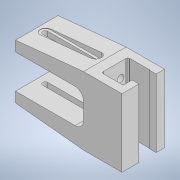
# Autodesk Inventor part: Z Belt 2
Saved by Autodesk Inventor 2022 (Build 260153000, 153)
## iProperties
Created: 2022-02-24
Part Number: Z Belt 2
Material: Generic
Document SubType Name: Modeling
Designer: Nicoli
Density: 1 g/cm^3
Appearance: Default
Author: Nicoli
Autodesk Inventor part; units mm, degrees
ref_plane "YZ Plane" through (0, 0, 0) normal (1, 0, 0) x (0, 1, 0)
ref_plane "XZ Plane" through (0, 0, 0) normal (0, 1, 0) x (-1, 0, 0)
ref_plane "XY Plane" through (0, 0, 0) normal (0, 0, 1) x (1, 0, 0)
sketch "Sketch1" plane through (0, 0, 0) normal (0, 0, 1) x (1, 0, 0)
  line L0 (-40, 0) -> (0, 0)
  line L1 (0, 0) -> (0, -20)
  line L2 (0, -20) -> (-40, -20)
  line L3 (-40, -20) -> (-40, -26)
  line L4 (-40, -26) -> (0, -30)
  line L5 (0, -30) -> (6, -30)
  line L6 (6, -30) -> (6, 10)
  line L7 (6, 10) -> (0, 10)
  line L8 (0, 10) -> (-40, 6)
  line L9 (-40, 6) -> (-40, 0)
  dimension "d0" = 6
  dimension "d1" = 40
  dimension "d2" = 20
  dimension "d3" = 40
  constraints: 20 end point, 5 equal length, 3 vertical, 2 horizontal, 2 perpendicular, 1 coincident, 1 parallel, 1 point on line
  measures "d0" distance of L8.end L0.start
  measures "d1" distance of L0.start L0.end
  measures "d2" distance of L0.end L1.end
  measures "d3" distance of L5.end L6.end
extrude "Extrusion1" add sketch "Sketch1" along normal blind 25
sketch "Sketch2" plane through (6, -30, 0) normal (1, 0, 0) x (0, 0, -1)
  line L0 (0, 40) -> (-25, 40) projected
  line L1 (0, 0) -> (-25, 0) projected
  line L2 (-25, 40) -> (-20, 40)
  line L3 (-20, 40) -> (-20, 0)
  line L4 (-20, 0) -> (-25, 0)
  line L5 (-25, 0) -> (-25, 40)
  line L6 (0, 0) -> (-5, 0)
  line L7 (-5, 0) -> (-5, 40)
  line L8 (-5, 40) -> (0, 40)
  line L9 (0, 40) -> (0, 0)
  circle A0 centre (-9, 8.6346) radius 1.7
  line L10 (-2.5, 11.8846) -> (-2.5, 5.3846)
  point P0 (0, 30)
  point P1 (-25, 0)
  point P2 (-5, 0)
  dimension "d6" = 5
  dimension "d7" = 5
  dimension "d30" = 4
  dimension "d31" = 8.6346
  constraints: 16 end point, 3 horizontal, 3 parallel, 2 point on line, 1 centre point, 1 perpendicular, 1 vertical, 3 other
  measures "d6" distance of L3.end L4.end
  measures "d7" distance of L8.start L8.end
  measures "d31" distance from line of L1 A0.centre
extrude "Extrusion2" add sketch "Sketch2" along normal blind 16.6 contours L9 L1 L7 L0 | L3 L1 L5 L0
hole "Hole2" at (6, -21.3654, 9) direction (-1, 0, 0) diameter 4 depth 6
sketch "Sketch3" plane through (0, 0, 0) normal (0, 0, -1) x (-1, 0, 0)
  line L0 (0, 0) -> (0, -20) projected
  arc A0 (0, -15) -> (5, -20) centre (5, -15) ccw
  arc A1 (5, 0) -> (0, -5) centre (5, -5) ccw
  line L1 (0, -20) -> (40, -20) projected
  line L2 (40, 0) -> (0, 0) projected
  dimension "d27" = 5
  constraints: 4 point on circle, 4 point on line, 4 tangent, 2 centre point, 1 equal radius
  measures "d27" radius of A0
extrude "Extrusion3" add sketch "Sketch3" against normal up to surface (25 mm away)
sketch "Sketch4" plane through (0, 10, 25) normal (0, 1, 0) x (1, 0, 0)
  line L0 (-5, 12.5) -> (-35, 12.5) construction
  line L1 (-5, 9.5) -> (-35, 9.5)
  line L2 (-35, 15.5) -> (-5, 15.5)
  arc A0 (-5, 9.5) -> (-5, 15.5) centre (-5, 12.5) ccw
  arc A1 (-35, 15.5) -> (-35, 9.5) centre (-35, 12.5) ccw
  line L3 (-40, 25) -> (-40, 0) projected
  line L4 (0, 25) -> (0, 0) projected
  point P0 (-20, 12.5)
  point P1 (0, 12.5)
  dimension "d32" = 3
  dimension "d33" = 5
  dimension "d34" = 5
  constraints: 8 end point, 4 point on circle, 4 tangent, 2 centre point, 2 midpoint, 1 horizontal, 1 parallel, 1 point on line
  measures "d32" radius of A1
  measures "d33" distance of point (0, 12.5) L0.start
  measures "d34" distance from line of L3 L0.end
extrude "Extrusion4" cut sketch "Sketch4" against normal blind 4
sketch "Sketch5" plane through (0, 6, 25) normal (0, 1, 0) x (1, 0, 0)
  line L0 (-5, 12.5) -> (-35, 12.5) construction
  line L1 (-5, 14) -> (-35, 14)
  line L2 (-35, 11) -> (-5, 11)
  arc A0 (-5, 11) -> (-5, 14) centre (-5, 12.5) ccw
  arc A1 (-35, 14) -> (-35, 11) centre (-35, 12.5) ccw
  line L3 (-5, 9.5) -> (-35, 9.5) projected
  arc A2 (-5, 9.5) -> (-5, 15.5) centre (-5, 12.5) ccw projected
  line L4 (-35, 15.5) -> (-5, 15.5) projected
  arc A3 (-35, 15.5) -> (-35, 9.5) centre (-35, 12.5) ccw projected
  point P0 (0, 25)
  point P1 (-20, 12.5)
  dimension "d37" = 1.5
  constraints: 8 end point, 4 point on circle, 4 tangent, 2 centre point, 2 coincident, 1 horizontal, 1 midpoint, 1 parallel
  measures "d37" radius of A1
extrude "Extrusion5" cut sketch "Sketch5" against normal blind 10.75 contours A0 L2 A1 L1
ref_plane "Work Plane1" through (-40, -10, 25) normal (0, 1, 0) x (1, 0, 0)
mirror "Mirror1" about plane through (-40, -10, 25) normal (0, 1, 0) of "Extrusion4", "Extrusion5", "Hole2"
sketch "Sketch6" plane through (6, -30, 20) normal (0, 0, -1) x (-1, 0, 0)
  line L0 (0, 40) -> (0, 0) projected
  line L1 (0, 40) -> (-16.6, 40) projected
  line L2 (-16.6, 0) -> (-16.6, 40) projected
  line L3 (0, 0) -> (-16.6, 0) projected
  line L4 (-16.6, 40) -> (-16.6, 0) projected
  line L5 (0, 0) -> (-16.6, 0) projected
  line L6 (-16.6, 40) -> (-12.6, 40)
  line L7 (-12.6, 40) -> (-12.6, 0)
  line L8 (-12.6, 0) -> (-16.6, 0)
  line L9 (-16.6, 0) -> (-16.6, 40)
  point P0 (6, 30)
  dimension "d40" = 4
  constraints: 8 end point, 2 parallel, 1 horizontal, 1 perpendicular, 1 point on line
  measures "d40" distance of L7.end L8.end
extrude "Extrusion6" add sketch "Sketch6" along normal blind 5 contours L7 L3 L2 L1
thicken "Thicken1" operation add thickness 0.1 both sides no extend neighbours yes toward (0, 0, 1) faces at (14.4, -3.3333, 20) (11.5333, -3.3333, 5)
sketch "Sketch7" plane through (0, 10, 25) normal (0, 1, 0) x (1, 0, 0)
  line L0 (6, 20.1) -> (6, 4.9) projected
  line L1 (5.8, 5.9) -> (6, 5.9)
  line L2 (6, 5.9) -> (6, 19.1)
  line L3 (6, 19.1) -> (5.8, 19.1)
  line L4 (5.8, 19.1) -> (5.8, 5.9)
  line L5 (6, 20.1) -> (22.6, 20.1) projected
  line L6 (7, 20.1) -> (18.6, 20.1)
  line L7 (18.6, 20.1) -> (18.6, 20.3)
  line L8 (18.6, 20.3) -> (7, 20.3)
  line L9 (7, 20.3) -> (7, 20.1)
  line L10 (6, 4.9) -> (18.6, 4.9) projected
  line L11 (7, 4.9) -> (17.6, 4.9)
  line L12 (17.6, 4.9) -> (17.6, 4.7)
  line L13 (17.6, 4.7) -> (7, 4.7)
  line L14 (7, 4.7) -> (7, 4.9)
  line L15 (18.6, 4.9) -> (18.6, 10) projected
  point P0 (0, 25)
  point P1 (6, 5.9)
  dimension "d45" = 1
  dimension "d46" = 1
  dimension "d47" = 0.2
  dimension "d48" = 0.2
  dimension "d49" = 1
  dimension "d50" = 1
  dimension "d51" = 0.2
  constraints: 24 end point, 6 parallel, 4 point on line, 3 horizontal, 3 perpendicular, 1 collinear
  measures "d45" distance between parallel lines of L15 L12
  measures "d46" distance between parallel lines of L0 L14
  measures "d47" distance of L13.end L11.start
  measures "d48" distance between parallel lines of L2 L4
  measures "d49" distance between parallel lines of L1 L10
  measures "d50" distance between parallel lines of L3 L5
  measures "d51" distance of L8.end L6.start
extrude "Extrusion7" cut sketch "Sketch7" against normal through all
body "Solid1"
